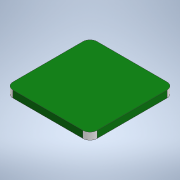
# Autodesk Inventor part: pcbe
Saved by Autodesk Inventor 2022.3 (Build 263350000, 350)
## iProperties
Created: 2022-12-14
Part Number: pcbe
Material: Generic
Document SubType Name: Modeling
Designer: komputer
Density: 1 g/cm^3
Appearance: Default
Author: komputer
Autodesk Inventor part; units mm, degrees
ref_plane "YZ Plane" through (0, 0, 0) normal (1, 0, 0) x (0, 1, 0)
ref_plane "XZ Plane" through (0, 0, 0) normal (0, 1, 0) x (-1, 0, 0)
ref_plane "XY Plane" through (0, 0, 0) normal (0, 0, 1) x (1, 0, 0)
sketch "Sketch1" plane through (0, 0, 0) normal (0, 1, 0) x (-1, 0, 0)
  line L0 (4.1296, 5.0085) -> (-19.8704, 5.0085)
  line L1 (-19.8704, 5.0085) -> (-19.8704, -18.9915)
  line L2 (-19.8704, -18.9915) -> (4.1296, -18.9915)
  line L3 (4.1296, -18.9915) -> (4.1296, 5.0085)
  point P0 (0, 0)
  dimension "d0" = 24
  dimension "d1" = 24
  constraints: 8 end point, 2 parallel, 1 horizontal, 1 perpendicular
  measures "d0" distance of L2.end L1.end
  measures "d1" distance of L1.end L0.end
extrude "Extrusion1" add sketch "Sketch1" along normal blind 2
fillet "Fillet1" radius 2 4 edges at (19.8704, 1, 5.0085) (19.8704, 1, -18.9915) (-4.1296, 1, -18.9915) (-4.1296, 1, 5.0085)
body "Solid1"
